Shoe Hanger (Autodesk Fusion 360 design; units mm, degrees)
Autodesk Fusion 360 part; units mm, degrees
note: some values were not read from the file. Set by a fixed rule: which sketch regions a step uses.
sketch "Sketch 1" plane through (0, 0, 0) normal (0, 1, 0) x (-1, 0, 0)
  line L0 (0.207, 14.4246) -> (-14.793, 14.4246)
  line L1 (0.207, 64.4246) -> (0.207, 14.4246)
  line L2 (-14.793, 14.4246) -> (-14.793, 64.4246)
  line L3 (-14.793, 64.4246) -> (0.207, 64.4246)
  line L4 (-92.925, 5.6402) -> (-78.1529, 8.2449)
  line L5 (-78.1529, 8.2449) -> (-89.7874, 74.227)
  line L6 (-104.5595, 71.6223) -> (-92.925, 5.6402)
  line L7 (-89.7874, 74.227) -> (-104.5595, 71.6223)
  circle A0 centre (-94.793, 59.4246) radius 4
  circle A1 centre (-87.7399, 19.4246) radius 4
  line L8 (0.207, 4.4246) -> (-114.793, 4.4246)
  line L9 (-114.793, 4.4246) -> (-114.793, 74.4246)
  line L10 (-114.793, 74.4246) -> (0.207, 74.4246)
  line L11 (0.207, 74.4246) -> (0.207, 4.4246)
  line L12 (0.207, 74.4246) -> (10, 74.4246)
  line L13 (10, 74.4246) -> (10, 44.4246)
  line L14 (10, 44.4246) -> (0.207, 44.4246)
  line L15 (0.207, 44.4246) -> (0.207, 74.4246)
  line L16 (-24.793, 67.4246) -> (-104.793, 67.4246)
  line L17 (-104.793, 67.4246) -> (-104.793, 51.4246)
  line L18 (-104.793, 51.4246) -> (-24.793, 51.4246)
  line L19 (-24.793, 51.4246) -> (-24.793, 67.4246)
  line L20 (-24.793, 27.4246) -> (-104.793, 27.4246)
  line L21 (-104.793, 27.4246) -> (-104.793, 11.4246)
  line L22 (-104.793, 11.4246) -> (-24.793, 11.4246)
  line L23 (-24.793, 11.4246) -> (-24.793, 27.4246)
  line L24 (-24.793, 51.4246) -> (-104.793, 51.4246)
  line L25 (-104.793, 51.4246) -> (-104.793, 59.4246)
  line L26 (-104.793, 59.4246) -> (-24.793, 59.4246)
  line L27 (-24.793, 59.4246) -> (-24.793, 51.4246)
  line L28 (-24.793, 11.4246) -> (-104.793, 11.4246)
  line L29 (-104.793, 11.4246) -> (-104.793, 19.4246)
  line L30 (-104.793, 19.4246) -> (-24.793, 19.4246)
  line L31 (-24.793, 19.4246) -> (-24.793, 11.4246)
  circle A2 centre (-30.793, 59.4246) radius 4
  circle A3 centre (-40.3644, 59.4246) radius 4
  circle A4 centre (-49.9359, 59.4246) radius 4
  circle A5 centre (-59.5073, 59.4246) radius 4
  circle A6 centre (-69.0787, 59.4246) radius 4
  circle A7 centre (-78.6501, 59.4246) radius 4
  circle A8 centre (-88.2216, 59.4246) radius 4
  circle A9 centre (-97.793, 59.4246) radius 4
  circle A10 centre (-30.793, 19.4246) radius 4
  circle A11 centre (-40.3644, 19.4246) radius 4
  circle A12 centre (-49.9359, 19.4246) radius 4
  circle A13 centre (-59.5073, 19.4246) radius 4
  circle A14 centre (-69.0787, 19.4246) radius 4
  circle A15 centre (-78.6501, 19.4246) radius 4
  circle A16 centre (-88.2216, 19.4246) radius 4
  circle A17 centre (-97.793, 19.4246) radius 4
  point P0 (-97.1734, 72.9246)
  dimension "d9" = 15
  dimension "d10" = 50
  dimension "d11" = 15
  dimension "d12" = 67
  dimension "d13" = 8
  dimension "d14" = 7.5
  dimension "d15" = 8
  dimension "d17" = 7.5
  dimension "d18" = 40
  dimension "d19" = 13.5
  dimension "d22" = 10
  dimension "d23" = 10
  dimension "d24" = 80
  dimension "d25" = 100
  dimension "d27" = 30
  dimension "d28" = 80
  dimension "d29" = 16
  dimension "d30" = 10
  dimension "d31" = 80
  dimension "d32" = 16
  dimension "d33" = 10
  dimension "d35" = 10
  dimension "d36" = 8
  dimension "d37" = 8
  dimension "d38" = 7
  dimension "d39" = 8
  dimension "d42" = -67
  dimension "d43" = 0
  dimension "d44" = 6
  dimension "d45" = 8
  dimension "d46" = 6
  dimension "d49" = -67
  dimension "d50" = 0
  constraint horizontal L3
  constraint horizontal L0
  constraint vertical L1
  constraint vertical L2
  constraint parallel L5 L6
  constraint parallel L4 L7
  constraint perpendicular L5 L7
  constraint midpoint L7 P0
  constraint horizontal L8
  constraint vertical L9
  constraint horizontal L10
  constraint vertical L11
  constraint horizontal L12
  constraint vertical L13
  constraint horizontal L14
  constraint vertical L15
  constraint horizontal L16
  constraint vertical L17
  constraint horizontal L18
  constraint vertical L19
  constraint horizontal L20
  constraint vertical L21
  constraint horizontal L22
  constraint vertical L23
  constraint horizontal L24
  constraint vertical L25
  constraint horizontal L26
  constraint vertical L27
  constraint midpoint L17 L25.end
  constraint horizontal L28
  constraint vertical L29
  constraint horizontal L30
  constraint vertical L31
  constraint midpoint L21 L29.end
  constraint coincident L26 A2.centre
  constraint coincident L30 A10.centre
  constraint midpoint L1 L11
  measures "d9" distance of L0.start L0.end
  measures "d10" distance of L0.start L1.start
  measures "d11" distance of L4.end L4.start
  measures "d12" distance of L4.end L5.end
  measures "d13" diameter of A0
  measures "d14" distance of L5 A0.centre
  measures "d15" diameter of A1
  measures "d17" distance of L5 A1.centre
  measures "d18" vertical distance of A0.centre A1.centre
  measures "d19" vertical distance of A0.centre P0
  measures "d22" distance of L3 L10
  measures "d23" distance of L0 L8
  measures "d24" distance of L2 A0.centre
  measures "d25" distance of L2 L9
  measures "d27" distance of L12.end L13.end
  measures "d28" distance of L16.start L16.end
  measures "d29" distance of L16.start L18.end
  measures "d30" distance of L9 L17
  measures "d31" distance of L20.start L20.end
  measures "d32" distance of L20.start L22.end
  measures "d33" distance of L9 L21
  measures "d35" angle of L2 L5
  measures "d36" distance of A0.centre L16
  measures "d37" distance of A1.centre L20
  measures "d38" distance of L10 L16
  measures "d39" diameter of A2
  measures "d44" distance of L19 A2.centre
  measures "d45" diameter of A10
  measures "d46" distance of L23 A10.centre
extrude "Extrude3" add sketch "Sketch 1" along normal blind 200 contours L0 L1 L2 L3 L11 L15 | L4 L5 L6 L22 L28 | L5 L6 A1 L22 L28 L30 A15 A16 A17 | L6 L30 A17 | L5 L30 A15 | L6 L30 A17 | L5 L6 A1 L20 L30 A15 A16 A17 | L5 L30 A15 | A1 L30 A16 | A1 L30 A16 | L5 L6 L18 L20 L24 | L5 L6 A0 L18 L24 L26 A8 A9 | L5 L6 A0 L16 L26 A8 A9 | L5 A0 L26 A8 | L5 L6 L7 L16 | A0 L26 A9 | A0 L26 A9 | L5 A0 L26 A8 picked at (-94.3244, 19.2578) picked at (-81.7956, 19.242) picked at (-94.3265, 19.6077) picked at (-81.7939, 19.6192) picked at (-91.9756, 20.1938) picked at (-91.9756, 18.6555) picked at (-99.7654, 59.8073) picked at (-99.7654, 59.042) makes body 1 at (14.793, 66.6667, 31.0913) makes body 2 at (100.6813, 66.6667, 49.6282)
extrude "Extrude4" add sketch "Sketch 1" along normal blind 10 separate body contours L0 L2 L3 L8 L9 L10 L11 L15 | L1 L11 L12 L13 L14 L15 | L4 L5 L6 L22 L28 | L6 L21 L22 L28 L29 L30 A17 | L5 L6 A1 L22 L28 L30 A15 A16 A17 | L5 L22 L23 L28 L30 L31 A10 A11 A12 A13 A14 A15 | L6 L30 A17 | L6 L30 A17 | L5 L30 A15 | L5 L30 A15 | L6 L30 A17 | L6 L30 A17 | L6 L20 L21 L30 A17 | L5 L6 A1 L20 L30 A15 A16 A17 | L5 L30 A15 | L5 L30 A15 | L5 L20 L23 L30 A10 A11 A12 A13 A14 A15 | A1 L30 A16 | A1 L30 A16 | A1 L30 A16 | A1 L30 A16 | L30 A14 | L30 A14 | L30 A10 | L30 A10 | L5 L6 L18 L20 L24 | A1 L30 A16 | A1 L30 A16 | L6 L17 L18 L24 L25 L26 | L5 L6 A0 L18 L24 L26 A8 A9 | L5 L18 L19 L24 L26 L27 A2 A3 A4 A5 A6 A7 A8 | L30 A13 | L30 A13 | L30 A11 | L30 A11 | L6 L16 L17 L26 | L5 L6 A0 L16 L26 A8 A9 | L5 A0 L26 A8 | L5 L26 A8 | L5 L6 L7 L16 | A0 L26 A9 | A0 L26 A9 | L5 A0 L26 A8 | L5 L26 A8 | A0 L26 A8 | A0 L26 A8 A9 | L5 L16 L19 L26 A2 A3 A4 A5 A6 A7 A8 | L30 A12 | L30 A12 | A0 L26 A9 | A0 L26 A9 | A0 L26 A8 A9 | A0 L26 A8 | L26 A7 | L26 A7 | L26 A2 | L26 A2 | L26 A6 | L26 A6 | L26 A3 | L26 A3 | L26 A5 | L26 A5 | L26 A4 | L26 A4 makes body 3
extrude "Extrude5" cut sketch "Sketch 1" along normal blind 4 from surface at 6 contours L6 L16 L17 L26 | L5 L6 A0 L16 L26 A8 A9 | L5 A0 L26 A8 | L5 L26 A8 | A0 L26 A9 | A0 L26 A9 | L5 A0 L26 A8 | L5 L26 A8 | A0 L26 A8 | L5 L16 L19 L26 A2 A3 A4 A5 A6 A7 A8 | A0 L26 A9 | A0 L26 A9 | A0 L26 A8 A9 | A0 L26 A8 | L26 A7 | L26 A7 | L26 A2 | L26 A2 | L26 A6 | L26 A6 | L26 A3 | L26 A3 | L26 A5 | L26 A5 | L26 A4 | L26 A4 picked at (-92.8229, 61.5231) bodies 3
extrude "Extrude6" cut sketch "Sketch 1" along normal blind 4 from surface at 6 contours L6 L30 A17 | L6 L30 A17 | L5 L30 A15 | L5 L30 A15 | L6 L30 A17 | L6 L30 A17 | L6 L20 L21 L30 A17 | L5 L6 A1 L20 L30 A15 A16 A17 | L5 L30 A15 | L5 L30 A15 | L5 L20 L23 L30 A10 A11 A12 A13 A14 A15 | A1 L30 A16 | A1 L30 A16 | A1 L30 A16 | L30 A14 | L30 A14 | L30 A10 | L30 A10 | A1 L30 A16 | A1 L30 A16 | L30 A13 | L30 A13 | L30 A11 | L30 A11 | L30 A12 | L30 A12 picked at (-91.9756, 20.1938) picked at (-91.9756, 18.6555) picked at (-83.9859, 20.1938) picked at (-89.2213, 19.2421) picked at (-89.2213, 19.6072) bodies 3
hidden bodies 1 2
